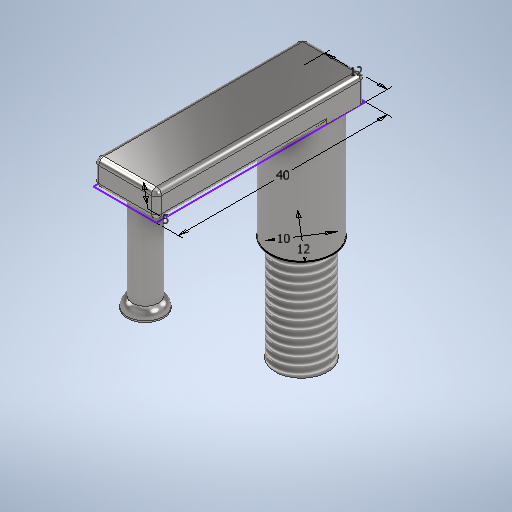
# Autodesk Inventor part: clamp
Saved by Autodesk Inventor 2025 (Build 290162000, 162)
## iProperties
Created: 2025-07-13
Part Number: clamp
Material: Steel, Carbon
Document SubType Name: Modeling
Designer: dr1e22
Density: 7.85 g/cm^3
Appearance: Semi-Polished
Mass: 53.5159 g
Surface Area: 31.8235 cm^2
Volume: 6.81731 cm^3
Author: dr1e22
Autodesk Inventor part; units mm, degrees
ref_plane "YZ Plane" through (0, 0, 0) normal (1, 0, 0) x (0, 1, 0)
ref_plane "XZ Plane" through (0, 0, 0) normal (0, 1, 0) x (-1, 0, 0)
ref_plane "XY Plane" through (0, 0, 0) normal (0, 0, 1) x (1, 0, 0)
sketch "Sketch1" plane through (0, 0, 0) normal (0, 1, 0) x (-1, 0, 0)
  circle A0 centre (0, 0) radius 5
  circle A1 centre (0, 0) radius 6
  dimension "d0" = 10
  dimension "d1" = 12
  constraints: 2 centre point, 2 coincident
  measures "d0" diameter of A0
  measures "d1" diameter of A1
extrude "Extrusion1" add sketch "Sketch1" against normal blind 20 contours A0
extrude "Extrusion2" add sketch "Sketch1" along normal blind 22 contours A0 | A1
sketch "Sketch2" plane through (0, 22, 0) normal (0, 1, 0) x (1, 0, 0)
  line L0 (-6.0998, -33.6689) -> (5.9002, -33.6689)
  line L1 (5.9002, -33.6689) -> (5.9002, 6.3311)
  line L2 (5.9002, 6.3311) -> (-6.0998, 6.3311)
  line L3 (-6.0998, 6.3311) -> (-6.0998, -33.6689)
  circle A0 centre (-0.0998, -29.7677) radius 2.5
  point P0 (0, 0)
  dimension "d8" = 12
  dimension "d9" = 40
  dimension "d15" = 5
  constraints: 8 end point, 2 parallel, 1 centre point, 1 horizontal, 1 perpendicular
  measures "d8" distance of L2.end L1.end
  measures "d9" distance of L1.end L0.end
  measures "d15" diameter of A0
extrude "Extrusion3" add sketch "Sketch2" along normal blind 5 contours L3 L2 L1 L0 | A0
fillet "Fillet1" radius 1 11 edges at (5.9002, 27, 13.6689) (5.9002, 22, 17.3793) (5.9002, 24.5, -6.3311) (-0.0998, 27, -6.3311) (-6.0998, 27, 13.6689) (-0.0998, 27, 33.6689) (-6.0998, 24.5, 33.6689) (-6.0998, 22, 13.6689) (-6.0998, 24.5, -6.3311) (-0.0998, 22, 33.6689) (5.9002, 24.5, 33.6689)
thread "Thread1" size "M10x1.5" class "6g" standard "ANSI Metric M Profile" full length
extrude "Extrusion4" add sketch "Sketch2" against normal blind 17 contours A0
sketch "Sketch3" plane through (-0.0998, 5, 29.7677) normal (0, -1, 0) x (1, 0, 0)
  circle A0 centre (0, 0) radius 3.5
  point P0 (0.0998, -29.7677)
  dimension "d18" = 7
  constraints: 1 centre point
  measures "d18" diameter of A0
extrude "Extrusion5" add sketch "Sketch3" along normal blind 2
fillet "Fillet2" radius 2 1 edges at (-3.5998, 5, 29.7677)
sketch "Sketch4" plane through (-0.0998, 3, 29.7677) normal (0, -1, 0) x (1, 0, 0)
  point P0 (0.0998, -29.7677)
body "Solid1"
